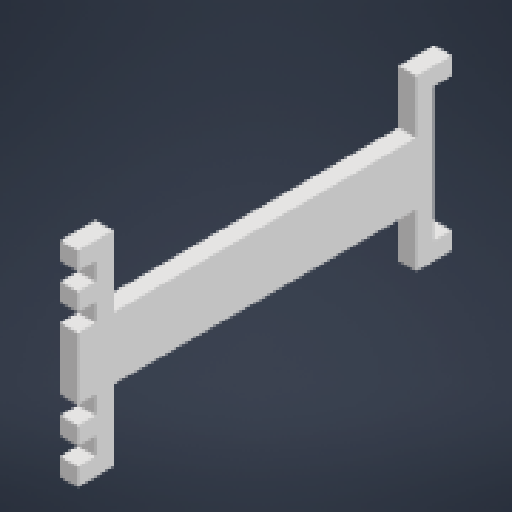
# Autodesk Inventor part: FootConnector
Saved by Autodesk Inventor 2027 (Build 310192000, 192)
## iProperties
Created: 2026-04-15
Part Number: FootConnector
Material: Generic
Document SubType Name: Modeling
Designer: Tueha
Density: 1 g/cm^3
Appearance: Default
Author: Tueha
Autodesk Inventor part; units mm, degrees
ref_plane "YZ Plane" through (0, 0, 0) normal (1, 0, 0) x (0, 1, 0)
ref_plane "XZ Plane" through (0, 0, 0) normal (0, 1, 0) x (-1, 0, 0)
ref_plane "XY Plane" through (0, 0, 0) normal (0, 0, 1) x (1, 0, 0)
sketch "Sketch1" plane through (0, 0, 0) normal (0, 0, 1) x (1, 0, 0)
  line L0 (316.5108, 23.0377) -> (310.3108, 23.0377) projected
  line L1 (316.5108, 39.9377) -> (316.5108, 23.0377) projected
  line L2 (316.5108, 39.9377) -> (24.9108, 39.9377) projected
  line L3 (24.9108, 39.9377) -> (24.9108, 45.9377) projected
  line L4 (24.9108, 45.9377) -> (316.5108, 45.9377) projected
  line L5 (316.5108, 62.8377) -> (316.5108, 45.9377) projected
  line L6 (301.1069, 62.8377) -> (316.5108, 62.8377) projected
  line L7 (295.9108, 65.8377) -> (301.1069, 62.8377) projected
  line L8 (295.9108, 62.8377) -> (295.9108, 65.8377) projected
  arc A0 (293.9108, 62.8377) -> (295.9108, 62.8377) centre (294.9108, 62.8377) ccw projected
  line L9 (293.9108, 65.8377) -> (293.9108, 62.8377) projected
  line L10 (288.7146, 62.8377) -> (293.9108, 65.8377) projected
  line L11 (272.3069, 62.8377) -> (288.7146, 62.8377) projected
  line L12 (267.1108, 65.8377) -> (272.3069, 62.8377) projected
  line L13 (267.1108, 62.8377) -> (267.1108, 65.8377) projected
  arc A1 (265.1108, 62.8377) -> (267.1108, 62.8377) centre (266.1108, 62.8377) ccw projected
  line L14 (265.1108, 65.8377) -> (265.1108, 62.8377) projected
  line L15 (259.9146, 62.8377) -> (265.1108, 65.8377) projected
  line L16 (243.5069, 62.8377) -> (259.9146, 62.8377) projected
  line L17 (238.3108, 65.8377) -> (243.5069, 62.8377) projected
  line L18 (238.3108, 62.8377) -> (238.3108, 65.8377) projected
  arc A2 (236.3108, 62.8377) -> (238.3108, 62.8377) centre (237.3108, 62.8377) ccw projected
  line L19 (236.3108, 65.8377) -> (236.3108, 62.8377) projected
  line L20 (231.1146, 62.8377) -> (236.3108, 65.8377) projected
  line L21 (214.7069, 62.8377) -> (231.1146, 62.8377) projected
  line L22 (209.5108, 65.8377) -> (214.7069, 62.8377) projected
  line L23 (209.5108, 62.8377) -> (209.5108, 65.8377) projected
  arc A3 (207.5108, 62.8377) -> (209.5108, 62.8377) centre (208.5108, 62.8377) ccw projected
  line L24 (207.5108, 65.8377) -> (207.5108, 62.8377) projected
  line L25 (202.3146, 62.8377) -> (207.5108, 65.8377) projected
  line L26 (185.9069, 62.8377) -> (202.3146, 62.8377) projected
  line L27 (180.7108, 65.8377) -> (185.9069, 62.8377) projected
  line L28 (180.7108, 62.8377) -> (180.7108, 65.8377) projected
  arc A4 (178.7108, 62.8377) -> (180.7108, 62.8377) centre (179.7108, 62.8377) ccw projected
  line L29 (178.7108, 65.8377) -> (178.7108, 62.8377) projected
  line L30 (173.5146, 62.8377) -> (178.7108, 65.8377) projected
  line L31 (157.1069, 62.8377) -> (173.5146, 62.8377) projected
  line L32 (151.9108, 65.8377) -> (157.1069, 62.8377) projected
  line L33 (151.9108, 62.8377) -> (151.9108, 65.8377) projected
  arc A5 (149.9108, 62.8377) -> (151.9108, 62.8377) centre (150.9108, 62.8377) ccw projected
  line L34 (149.9108, 65.8377) -> (149.9108, 62.8377) projected
  line L35 (144.7146, 62.8377) -> (149.9108, 65.8377) projected
  line L36 (128.3069, 62.8377) -> (144.7146, 62.8377) projected
  line L37 (123.1108, 65.8377) -> (128.3069, 62.8377) projected
  line L38 (123.1108, 62.8377) -> (123.1108, 65.8377) projected
  arc A6 (121.1108, 62.8377) -> (123.1108, 62.8377) centre (122.1108, 62.8377) ccw projected
  line L39 (121.1108, 65.8377) -> (121.1108, 62.8377) projected
  line L40 (115.9146, 62.8377) -> (121.1108, 65.8377) projected
  line L41 (99.5069, 62.8377) -> (115.9146, 62.8377) projected
  line L42 (94.3108, 65.8377) -> (99.5069, 62.8377) projected
  line L43 (94.3108, 62.8377) -> (94.3108, 65.8377) projected
  arc A7 (92.3108, 62.8377) -> (94.3108, 62.8377) centre (93.3108, 62.8377) ccw projected
  line L44 (92.3108, 65.8377) -> (92.3108, 62.8377) projected
  line L45 (87.1146, 62.8377) -> (92.3108, 65.8377) projected
  line L46 (70.7069, 62.8377) -> (87.1146, 62.8377) projected
  line L47 (65.5108, 65.8377) -> (70.7069, 62.8377) projected
  line L48 (65.5108, 62.8377) -> (65.5108, 65.8377) projected
  arc A8 (63.5108, 62.8377) -> (65.5108, 62.8377) centre (64.5108, 62.8377) ccw projected
  line L49 (63.5108, 65.8377) -> (63.5108, 62.8377) projected
  line L50 (58.3146, 62.8377) -> (63.5108, 65.8377) projected
  line L51 (41.9069, 62.8377) -> (58.3146, 62.8377) projected
  line L52 (36.7108, 65.8377) -> (41.9069, 62.8377) projected
  line L53 (36.7108, 62.8377) -> (36.7108, 65.8377) projected
  arc A9 (34.7108, 62.8377) -> (36.7108, 62.8377) centre (35.7108, 62.8377) ccw projected
  line L54 (34.7108, 65.8377) -> (34.7108, 62.8377) projected
  line L55 (29.5146, 62.8377) -> (34.7108, 65.8377) projected
  line L56 (13.1069, 62.8377) -> (29.5146, 62.8377) projected
  line L57 (7.9108, 65.8377) -> (13.1069, 62.8377) projected
  line L58 (7.9108, 62.8377) -> (7.9108, 65.8377) projected
  arc A10 (5.9108, 62.8377) -> (7.9108, 62.8377) centre (6.9108, 62.8377) ccw projected
  line L59 (5.9108, 65.8377) -> (5.9108, 62.8377) projected
  line L60 (0.7146, 62.8377) -> (5.9108, 65.8377) projected
  line L61 (-15.6931, 62.8377) -> (0.7146, 62.8377) projected
  line L62 (-20.8892, 65.8377) -> (-15.6931, 62.8377) projected
  line L63 (-20.8892, 62.8377) -> (-20.8892, 65.8377) projected
  arc A11 (-22.8892, 62.8377) -> (-20.8892, 62.8377) centre (-21.8892, 62.8377) ccw projected
  line L64 (-22.8892, 65.8377) -> (-22.8892, 62.8377) projected
  line L65 (-28.0854, 62.8377) -> (-22.8892, 65.8377) projected
  line L66 (-44.4931, 62.8377) -> (-28.0854, 62.8377) projected
  line L67 (-49.6892, 65.8377) -> (-44.4931, 62.8377) projected
  line L68 (-49.6892, 62.8377) -> (-49.6892, 65.8377) projected
  arc A12 (-51.6892, 62.8377) -> (-49.6892, 62.8377) centre (-50.6892, 62.8377) ccw projected
  line L69 (-51.6892, 65.8377) -> (-51.6892, 62.8377) projected
  line L70 (-56.8854, 62.8377) -> (-51.6892, 65.8377) projected
  line L71 (-73.2931, 62.8377) -> (-56.8854, 62.8377) projected
  line L72 (-78.4892, 65.8377) -> (-73.2931, 62.8377) projected
  line L73 (-78.4892, 62.8377) -> (-78.4892, 65.8377) projected
  arc A13 (-80.4892, 62.8377) -> (-78.4892, 62.8377) centre (-79.4892, 62.8377) ccw projected
  line L74 (-80.4892, 65.8377) -> (-80.4892, 62.8377) projected
  line L75 (-85.6854, 62.8377) -> (-80.4892, 65.8377) projected
  line L76 (-102.0931, 62.8377) -> (-85.6854, 62.8377) projected
  line L77 (-107.2892, 65.8377) -> (-102.0931, 62.8377) projected
  line L78 (-107.2892, 62.8377) -> (-107.2892, 65.8377) projected
  arc A14 (-109.2892, 62.8377) -> (-107.2892, 62.8377) centre (-108.2892, 62.8377) ccw projected
  line L79 (-109.2892, 65.8377) -> (-109.2892, 62.8377) projected
  line L80 (-114.4854, 62.8377) -> (-109.2892, 65.8377) projected
  line L81 (-130.8931, 62.8377) -> (-114.4854, 62.8377) projected
  line L82 (-136.0892, 65.8377) -> (-130.8931, 62.8377) projected
  line L83 (-136.0892, 62.8377) -> (-136.0892, 65.8377) projected
  arc A15 (-138.0892, 62.8377) -> (-136.0892, 62.8377) centre (-137.0892, 62.8377) ccw projected
  line L84 (-138.0892, 65.8377) -> (-138.0892, 62.8377) projected
  line L85 (-143.2854, 62.8377) -> (-138.0892, 65.8377) projected
  line L86 (-159.6931, 62.8377) -> (-143.2854, 62.8377) projected
  line L87 (-164.8892, 65.8377) -> (-159.6931, 62.8377) projected
  line L88 (-164.8892, 62.8377) -> (-164.8892, 65.8377) projected
  arc A16 (-166.8892, 62.8377) -> (-164.8892, 62.8377) centre (-165.8892, 62.8377) ccw projected
  line L89 (-166.8892, 65.8377) -> (-166.8892, 62.8377) projected
  line L90 (-172.0854, 62.8377) -> (-166.8892, 65.8377) projected
  line L91 (-188.4931, 62.8377) -> (-172.0854, 62.8377) projected
  line L92 (-193.6892, 65.8377) -> (-188.4931, 62.8377) projected
  line L93 (-193.6892, 62.8377) -> (-193.6892, 65.8377) projected
  arc A17 (-195.6892, 62.8377) -> (-193.6892, 62.8377) centre (-194.6892, 62.8377) ccw projected
  line L94 (-195.6892, 65.8377) -> (-195.6892, 62.8377) projected
  line L95 (-200.8854, 62.8377) -> (-195.6892, 65.8377) projected
  line L96 (-217.2931, 62.8377) -> (-200.8854, 62.8377) projected
  line L97 (-222.4892, 65.8377) -> (-217.2931, 62.8377) projected
  line L98 (-222.4892, 62.8377) -> (-222.4892, 65.8377) projected
  arc A18 (-224.4892, 62.8377) -> (-222.4892, 62.8377) centre (-223.4892, 62.8377) ccw projected
  line L99 (-224.4892, 65.8377) -> (-224.4892, 62.8377) projected
  line L100 (-229.6854, 62.8377) -> (-224.4892, 65.8377) projected
  line L101 (-246.0931, 62.8377) -> (-229.6854, 62.8377) projected
  line L102 (-251.2892, 65.8377) -> (-246.0931, 62.8377) projected
  line L103 (-251.2892, 62.8377) -> (-251.2892, 65.8377) projected
  arc A19 (-253.2892, 62.8377) -> (-251.2892, 62.8377) centre (-252.2892, 62.8377) ccw projected
  line L104 (-253.2892, 65.8377) -> (-253.2892, 62.8377) projected
  line L105 (-258.4854, 62.8377) -> (-253.2892, 65.8377) projected
  line L106 (-258.4854, 62.8377) -> (-266.6892, 62.8377) projected
  line L107 (-266.6892, 23.0377) -> (-266.6892, 62.8377) projected
  line L108 (-244.0854, 23.0377) -> (-266.6892, 23.0377) projected
  line L109 (-238.8892, 20.0377) -> (-244.0854, 23.0377) projected
  line L110 (-238.8892, 23.0377) -> (-238.8892, 20.0377) projected
  arc A20 (-236.8892, 23.0377) -> (-238.8892, 23.0377) centre (-237.8892, 23.0377) ccw projected
  line L111 (-236.8892, 20.0377) -> (-236.8892, 23.0377) projected
  line L112 (-231.6931, 23.0377) -> (-236.8892, 20.0377) projected
  line L113 (-215.2854, 23.0377) -> (-231.6931, 23.0377) projected
  line L114 (-210.0892, 20.0377) -> (-215.2854, 23.0377) projected
  line L115 (-210.0892, 23.0377) -> (-210.0892, 20.0377) projected
  arc A21 (-208.0892, 23.0377) -> (-210.0892, 23.0377) centre (-209.0892, 23.0377) ccw projected
  line L116 (-208.0892, 20.0377) -> (-208.0892, 23.0377) projected
  line L117 (-202.8931, 23.0377) -> (-208.0892, 20.0377) projected
  line L118 (-186.4854, 23.0377) -> (-202.8931, 23.0377) projected
  line L119 (-181.2892, 20.0377) -> (-186.4854, 23.0377) projected
  line L120 (-181.2892, 23.0377) -> (-181.2892, 20.0377) projected
  arc A22 (-179.2892, 23.0377) -> (-181.2892, 23.0377) centre (-180.2892, 23.0377) ccw projected
  line L121 (-179.2892, 20.0377) -> (-179.2892, 23.0377) projected
  line L122 (-174.0931, 23.0377) -> (-179.2892, 20.0377) projected
  line L123 (-157.6854, 23.0377) -> (-174.0931, 23.0377) projected
  line L124 (-152.4892, 20.0377) -> (-157.6854, 23.0377) projected
  line L125 (-152.4892, 23.0377) -> (-152.4892, 20.0377) projected
  arc A23 (-150.4892, 23.0377) -> (-152.4892, 23.0377) centre (-151.4892, 23.0377) ccw projected
  line L126 (-150.4892, 20.0377) -> (-150.4892, 23.0377) projected
  line L127 (-145.2931, 23.0377) -> (-150.4892, 20.0377) projected
  line L128 (-128.8854, 23.0377) -> (-145.2931, 23.0377) projected
  line L129 (-123.6892, 20.0377) -> (-128.8854, 23.0377) projected
  line L130 (-123.6892, 23.0377) -> (-123.6892, 20.0377) projected
  arc A24 (-121.6892, 23.0377) -> (-123.6892, 23.0377) centre (-122.6892, 23.0377) ccw projected
  line L131 (-121.6892, 20.0377) -> (-121.6892, 23.0377) projected
  line L132 (-116.4931, 23.0377) -> (-121.6892, 20.0377) projected
  line L133 (-100.0854, 23.0377) -> (-116.4931, 23.0377) projected
  line L134 (-94.8892, 20.0377) -> (-100.0854, 23.0377) projected
  line L135 (-94.8892, 23.0377) -> (-94.8892, 20.0377) projected
  arc A25 (-92.8892, 23.0377) -> (-94.8892, 23.0377) centre (-93.8892, 23.0377) ccw projected
  line L136 (-92.8892, 20.0377) -> (-92.8892, 23.0377) projected
  line L137 (-87.6931, 23.0377) -> (-92.8892, 20.0377) projected
  line L138 (-71.2854, 23.0377) -> (-87.6931, 23.0377) projected
  line L139 (-66.0892, 20.0377) -> (-71.2854, 23.0377) projected
  line L140 (-66.0892, 23.0377) -> (-66.0892, 20.0377) projected
  arc A26 (-64.0892, 23.0377) -> (-66.0892, 23.0377) centre (-65.0892, 23.0377) ccw projected
  line L141 (-64.0892, 20.0377) -> (-64.0892, 23.0377) projected
  line L142 (-58.8931, 23.0377) -> (-64.0892, 20.0377) projected
  line L143 (-42.4854, 23.0377) -> (-58.8931, 23.0377) projected
  line L144 (-37.2892, 20.0377) -> (-42.4854, 23.0377) projected
  line L145 (-37.2892, 23.0377) -> (-37.2892, 20.0377) projected
  arc A27 (-35.2892, 23.0377) -> (-37.2892, 23.0377) centre (-36.2892, 23.0377) ccw projected
  line L146 (-35.2892, 20.0377) -> (-35.2892, 23.0377) projected
  line L147 (-30.0931, 23.0377) -> (-35.2892, 20.0377) projected
  line L148 (-13.6854, 23.0377) -> (-30.0931, 23.0377) projected
  line L149 (-8.4892, 20.0377) -> (-13.6854, 23.0377) projected
  line L150 (-8.4892, 23.0377) -> (-8.4892, 20.0377) projected
  arc A28 (-6.4892, 23.0377) -> (-8.4892, 23.0377) centre (-7.4892, 23.0377) ccw projected
  line L151 (-6.4892, 20.0377) -> (-6.4892, 23.0377) projected
  line L152 (-1.2931, 23.0377) -> (-6.4892, 20.0377) projected
  line L153 (15.1146, 23.0377) -> (-1.2931, 23.0377) projected
  line L154 (20.3108, 20.0377) -> (15.1146, 23.0377) projected
  line L155 (20.3108, 23.0377) -> (20.3108, 20.0377) projected
  arc A29 (22.3108, 23.0377) -> (20.3108, 23.0377) centre (21.3108, 23.0377) ccw projected
  line L156 (22.3108, 20.0377) -> (22.3108, 23.0377) projected
  line L157 (27.5069, 23.0377) -> (22.3108, 20.0377) projected
  line L158 (43.9146, 23.0377) -> (27.5069, 23.0377) projected
  line L159 (49.1108, 20.0377) -> (43.9146, 23.0377) projected
  line L160 (49.1108, 23.0377) -> (49.1108, 20.0377) projected
  arc A30 (51.1108, 23.0377) -> (49.1108, 23.0377) centre (50.1108, 23.0377) ccw projected
  line L161 (51.1108, 20.0377) -> (51.1108, 23.0377) projected
  line L162 (56.3069, 23.0377) -> (51.1108, 20.0377) projected
  line L163 (72.7146, 23.0377) -> (56.3069, 23.0377) projected
  line L164 (77.9108, 20.0377) -> (72.7146, 23.0377) projected
  line L165 (77.9108, 23.0377) -> (77.9108, 20.0377) projected
  arc A31 (79.9108, 23.0377) -> (77.9108, 23.0377) centre (78.9108, 23.0377) ccw projected
  line L166 (79.9108, 20.0377) -> (79.9108, 23.0377) projected
  line L167 (85.1069, 23.0377) -> (79.9108, 20.0377) projected
  line L168 (101.5146, 23.0377) -> (85.1069, 23.0377) projected
  line L169 (106.7108, 20.0377) -> (101.5146, 23.0377) projected
  line L170 (106.7108, 23.0377) -> (106.7108, 20.0377) projected
  arc A32 (108.7108, 23.0377) -> (106.7108, 23.0377) centre (107.7108, 23.0377) ccw projected
  line L171 (108.7108, 20.0377) -> (108.7108, 23.0377) projected
  line L172 (113.9069, 23.0377) -> (108.7108, 20.0377) projected
  line L173 (130.3146, 23.0377) -> (113.9069, 23.0377) projected
  line L174 (135.5108, 20.0377) -> (130.3146, 23.0377) projected
  line L175 (135.5108, 23.0377) -> (135.5108, 20.0377) projected
  arc A33 (137.5108, 23.0377) -> (135.5108, 23.0377) centre (136.5108, 23.0377) ccw projected
  line L176 (137.5108, 20.0377) -> (137.5108, 23.0377) projected
  line L177 (142.7069, 23.0377) -> (137.5108, 20.0377) projected
  line L178 (159.1146, 23.0377) -> (142.7069, 23.0377) projected
  line L179 (164.3108, 20.0377) -> (159.1146, 23.0377) projected
  line L180 (164.3108, 23.0377) -> (164.3108, 20.0377) projected
  arc A34 (166.3108, 23.0377) -> (164.3108, 23.0377) centre (165.3108, 23.0377) ccw projected
  line L181 (166.3108, 20.0377) -> (166.3108, 23.0377) projected
  line L182 (171.5069, 23.0377) -> (166.3108, 20.0377) projected
  line L183 (187.9146, 23.0377) -> (171.5069, 23.0377) projected
  line L184 (193.1108, 20.0377) -> (187.9146, 23.0377) projected
  line L185 (193.1108, 23.0377) -> (193.1108, 20.0377) projected
  arc A35 (195.1108, 23.0377) -> (193.1108, 23.0377) centre (194.1108, 23.0377) ccw projected
  line L186 (195.1108, 20.0377) -> (195.1108, 23.0377) projected
  line L187 (200.3069, 23.0377) -> (195.1108, 20.0377) projected
  line L188 (216.7146, 23.0377) -> (200.3069, 23.0377) projected
  line L189 (221.9108, 20.0377) -> (216.7146, 23.0377) projected
  line L190 (221.9108, 23.0377) -> (221.9108, 20.0377) projected
  arc A36 (223.9108, 23.0377) -> (221.9108, 23.0377) centre (222.9108, 23.0377) ccw projected
  line L191 (223.9108, 20.0377) -> (223.9108, 23.0377) projected
  line L192 (229.1069, 23.0377) -> (223.9108, 20.0377) projected
  line L193 (245.5146, 23.0377) -> (229.1069, 23.0377) projected
  line L194 (250.7108, 20.0377) -> (245.5146, 23.0377) projected
  line L195 (250.7108, 23.0377) -> (250.7108, 20.0377) projected
  arc A37 (252.7108, 23.0377) -> (250.7108, 23.0377) centre (251.7108, 23.0377) ccw projected
  line L196 (252.7108, 20.0377) -> (252.7108, 23.0377) projected
  line L197 (257.9069, 23.0377) -> (252.7108, 20.0377) projected
  line L198 (274.3146, 23.0377) -> (257.9069, 23.0377) projected
  line L199 (279.5108, 20.0377) -> (274.3146, 23.0377) projected
  line L200 (279.5108, 23.0377) -> (279.5108, 20.0377) projected
  arc A38 (281.5108, 23.0377) -> (279.5108, 23.0377) centre (280.5108, 23.0377) ccw projected
  line L201 (281.5108, 20.0377) -> (281.5108, 23.0377) projected
  line L202 (286.7069, 23.0377) -> (281.5108, 20.0377) projected
  line L203 (303.1146, 23.0377) -> (286.7069, 23.0377) projected
  line L204 (308.3108, 20.0377) -> (303.1146, 23.0377) projected
  line L205 (308.3108, 23.0377) -> (308.3108, 20.0377) projected
  arc A39 (310.3108, 23.0377) -> (308.3108, 23.0377) centre (309.3108, 23.0377) ccw projected
  line L206 (-237.2892, 33.9377) -> (-231.2892, 33.9377) projected
  line L207 (-231.2892, 33.9377) -> (-231.2892, 27.9377) projected
  line L208 (-231.2892, 27.9377) -> (-237.2892, 27.9377) projected
  line L209 (-237.2892, 27.9377) -> (-237.2892, 33.9377) projected
  line L210 (-237.2892, 51.9377) -> (-237.2892, 57.9377) projected
  line L211 (-237.2892, 57.9377) -> (-231.2892, 57.9377) projected
  line L212 (-231.2892, 57.9377) -> (-231.2892, 51.9377) projected
  line L213 (-231.2892, 51.9377) -> (-237.2892, 51.9377) projected
  line L214 (-179.6892, 33.9377) -> (-173.6892, 33.9377) projected
  line L215 (-173.6892, 33.9377) -> (-173.6892, 27.9377) projected
  line L216 (-173.6892, 27.9377) -> (-179.6892, 27.9377) projected
  line L217 (-179.6892, 27.9377) -> (-179.6892, 33.9377) projected
  line L218 (-179.6892, 51.9377) -> (-179.6892, 57.9377) projected
  line L219 (-179.6892, 57.9377) -> (-173.6892, 57.9377) projected
  line L220 (-173.6892, 57.9377) -> (-173.6892, 51.9377) projected
  line L221 (-173.6892, 51.9377) -> (-179.6892, 51.9377) projected
  line L222 (-122.0892, 33.9377) -> (-116.0892, 33.9377) projected
  line L223 (-116.0892, 33.9377) -> (-116.0892, 27.9377) projected
  line L224 (-116.0892, 27.9377) -> (-122.0892, 27.9377) projected
  line L225 (-122.0892, 27.9377) -> (-122.0892, 33.9377) projected
  line L226 (-122.0892, 51.9377) -> (-122.0892, 57.9377) projected
  line L227 (-122.0892, 57.9377) -> (-116.0892, 57.9377) projected
  line L228 (-116.0892, 57.9377) -> (-116.0892, 51.9377) projected
  line L229 (-116.0892, 51.9377) -> (-122.0892, 51.9377) projected
  line L230 (-64.4892, 33.9377) -> (-58.4892, 33.9377) projected
  line L231 (-58.4892, 33.9377) -> (-58.4892, 27.9377) projected
  line L232 (-58.4892, 27.9377) -> (-64.4892, 27.9377) projected
  line L233 (-64.4892, 27.9377) -> (-64.4892, 33.9377) projected
  line L234 (-64.4892, 51.9377) -> (-64.4892, 57.9377) projected
  line L235 (-64.4892, 57.9377) -> (-58.4892, 57.9377) projected
  line L236 (-58.4892, 57.9377) -> (-58.4892, 51.9377) projected
  line L237 (-58.4892, 51.9377) -> (-64.4892, 51.9377) projected
  line L238 (-6.8892, 33.9377) -> (-0.8892, 33.9377) projected
  line L239 (-0.8892, 33.9377) -> (-0.8892, 27.9377) projected
  line L240 (-0.8892, 27.9377) -> (-6.8892, 27.9377) projected
  line L241 (-6.8892, 27.9377) -> (-6.8892, 33.9377) projected
  line L242 (-6.8892, 51.9377) -> (-6.8892, 57.9377) projected
  line L243 (-6.8892, 57.9377) -> (-0.8892, 57.9377) projected
  line L244 (-0.8892, 57.9377) -> (-0.8892, 51.9377) projected
  line L245 (-0.8892, 51.9377) -> (-6.8892, 51.9377) projected
  line L246 (50.7108, 33.9377) -> (56.7108, 33.9377) projected
  line L247 (56.7108, 33.9377) -> (56.7108, 27.9377) projected
  line L248 (56.7108, 27.9377) -> (50.7108, 27.9377) projected
  line L249 (50.7108, 27.9377) -> (50.7108, 33.9377) projected
  line L250 (50.7108, 51.9377) -> (50.7108, 57.9377) projected
  line L251 (50.7108, 57.9377) -> (56.7108, 57.9377) projected
  line L252 (56.7108, 57.9377) -> (56.7108, 51.9377) projected
  line L253 (56.7108, 51.9377) -> (50.7108, 51.9377) projected
  line L254 (108.3108, 33.9377) -> (114.3108, 33.9377) projected
  line L255 (114.3108, 33.9377) -> (114.3108, 27.9377) projected
  line L256 (114.3108, 27.9377) -> (108.3108, 27.9377) projected
  line L257 (108.3108, 27.9377) -> (108.3108, 33.9377) projected
  line L258 (108.3108, 51.9377) -> (108.3108, 57.9377) projected
  line L259 (108.3108, 57.9377) -> (114.3108, 57.9377) projected
  line L260 (114.3108, 57.9377) -> (114.3108, 51.9377) projected
  line L261 (114.3108, 51.9377) -> (108.3108, 51.9377) projected
  line L262 (165.9108, 33.9377) -> (171.9108, 33.9377) projected
  line L263 (171.9108, 33.9377) -> (171.9108, 27.9377) projected
  line L264 (171.9108, 27.9377) -> (165.9108, 27.9377) projected
  line L265 (165.9108, 27.9377) -> (165.9108, 33.9377) projected
  line L266 (165.9108, 51.9377) -> (165.9108, 57.9377) projected
  line L267 (165.9108, 57.9377) -> (171.9108, 57.9377) projected
  line L268 (171.9108, 57.9377) -> (171.9108, 51.9377) projected
  line L269 (171.9108, 51.9377) -> (165.9108, 51.9377) projected
  line L270 (223.5108, 33.9377) -> (229.5108, 33.9377) projected
  line L271 (229.5108, 33.9377) -> (229.5108, 27.9377) projected
  line L272 (229.5108, 27.9377) -> (223.5108, 27.9377) projected
  line L273 (223.5108, 27.9377) -> (223.5108, 33.9377) projected
  line L274 (223.5108, 51.9377) -> (223.5108, 57.9377) projected
  line L275 (223.5108, 57.9377) -> (229.5108, 57.9377) projected
  line L276 (229.5108, 57.9377) -> (229.5108, 51.9377) projected
  line L277 (229.5108, 51.9377) -> (223.5108, 51.9377) projected
  line L278 (281.1108, 33.9377) -> (287.1108, 33.9377) projected
  line L279 (287.1108, 33.9377) -> (287.1108, 27.9377) projected
  line L280 (287.1108, 27.9377) -> (281.1108, 27.9377) projected
  line L281 (281.1108, 27.9377) -> (281.1108, 33.9377) projected
  line L282 (281.1108, 51.9377) -> (281.1108, 57.9377) projected
  line L283 (281.1108, 57.9377) -> (287.1108, 57.9377) projected
  line L284 (287.1108, 57.9377) -> (287.1108, 51.9377) projected
  line L285 (287.1108, 51.9377) -> (281.1108, 51.9377) projected
  line L286 (316.5108, -51.9623) -> (310.3108, -51.9623) projected
  line L287 (316.5108, -35.0623) -> (316.5108, -51.9623) projected
  line L288 (316.5108, -35.0623) -> (24.9108, -35.0623) projected
  line L289 (24.9108, -35.0623) -> (24.9108, -29.0623) projected
  line L290 (24.9108, -29.0623) -> (316.5108, -29.0623) projected
  line L291 (316.5108, -12.1623) -> (316.5108, -29.0623) projected
  line L292 (301.1069, -12.1623) -> (316.5108, -12.1623) projected
  line L293 (295.9108, -9.1623) -> (301.1069, -12.1623) projected
  line L294 (295.9108, -12.1623) -> (295.9108, -9.1623) projected
  arc A40 (293.9108, -12.1623) -> (295.9108, -12.1623) centre (294.9108, -12.1623) ccw projected
  line L295 (293.9108, -9.1623) -> (293.9108, -12.1623) projected
  line L296 (288.7146, -12.1623) -> (293.9108, -9.1623) projected
  line L297 (272.3069, -12.1623) -> (288.7146, -12.1623) projected
  line L298 (267.1108, -9.1623) -> (272.3069, -12.1623) projected
  line L299 (267.1108, -12.1623) -> (267.1108, -9.1623) projected
  arc A41 (265.1108, -12.1623) -> (267.1108, -12.1623) centre (266.1108, -12.1623) ccw projected
  line L300 (265.1108, -9.1623) -> (265.1108, -12.1623) projected
  line L301 (259.9146, -12.1623) -> (265.1108, -9.1623) projected
  line L302 (243.5069, -12.1623) -> (259.9146, -12.1623) projected
  line L303 (238.3108, -9.1623) -> (243.5069, -12.1623) projected
  line L304 (238.3108, -12.1623) -> (238.3108, -9.1623) projected
  arc A42 (236.3108, -12.1623) -> (238.3108, -12.1623) centre (237.3108, -12.1623) ccw projected
  line L305 (236.3108, -9.1623) -> (236.3108, -12.1623) projected
  line L306 (231.1146, -12.1623) -> (236.3108, -9.1623) projected
  line L307 (214.7069, -12.1623) -> (231.1146, -12.1623) projected
  line L308 (209.5108, -9.1623) -> (214.7069, -12.1623) projected
  line L309 (209.5108, -12.1623) -> (209.5108, -9.1623) projected
  arc A43 (207.5108, -12.1623) -> (209.5108, -12.1623) centre (208.5108, -12.1623) ccw projected
  line L310 (207.5108, -9.1623) -> (207.5108, -12.1623) projected
  line L311 (202.3146, -12.1623) -> (207.5108, -9.1623) projected
  line L312 (185.9069, -12.1623) -> (202.3146, -12.1623) projected
  line L313 (180.7108, -9.1623) -> (185.9069, -12.1623) projected
  line L314 (180.7108, -12.1623) -> (180.7108, -9.1623) projected
  arc A44 (178.7108, -12.1623) -> (180.7108, -12.1623) centre (179.7108, -12.1623) ccw projected
  line L315 (178.7108, -9.1623) -> (178.7108, -12.1623) projected
  line L316 (173.5146, -12.1623) -> (178.7108, -9.1623) projected
  line L317 (157.1069, -12.1623) -> (173.5146, -12.1623) projected
  line L318 (151.9108, -9.1623) -> (157.1069, -12.1623) projected
  line L319 (151.9108, -12.1623) -> (151.9108, -9.1623) projected
  arc A45 (149.9108, -12.1623) -> (151.9108, -12.1623) centre (150.9108, -12.1623) ccw projected
  line L320 (149.9108, -9.1623) -> (149.9108, -12.1623) projected
  line L321 (144.7146, -12.1623) -> (149.9108, -9.1623) projected
  line L322 (128.3069, -12.1623) -> (144.7146, -12.1623) projected
  line L323 (123.1108, -9.1623) -> (128.3069, -12.1623) projected
  line L324 (123.1108, -12.1623) -> (123.1108, -9.1623) projected
  arc A46 (121.1108, -12.1623) -> (123.1108, -12.1623) centre (122.1108, -12.1623) ccw projected
  line L325 (121.1108, -9.1623) -> (121.1108, -12.1623) projected
  line L326 (115.9146, -12.1623) -> (121.1108, -9.1623) projected
  line L327 (99.5069, -12.1623) -> (115.9146, -12.1623) projected
  line L328 (94.3108, -9.1623) -> (99.5069, -12.1623) projected
  line L329 (94.3108, -12.1623) -> (94.3108, -9.1623) projected
  arc A47 (92.3108, -12.1623) -> (94.3108, -12.1623) centre (93.3108, -12.1623) ccw projected
  line L330 (92.3108, -9.1623) -> (92.3108, -12.1623) projected
  line L331 (87.1146, -12.1623) -> (92.3108, -9.1623) projected
  line L332 (70.7069, -12.1623) -> (87.1146, -12.1623) projected
  line L333 (65.5108, -9.1623) -> (70.7069, -12.1623) projected
  line L334 (65.5108, -12.1623) -> (65.5108, -9.1623) projected
  arc A48 (63.5108, -12.1623) -> (65.5108, -12.1623) centre (64.5108, -12.1623) ccw projected
  line L335 (63.5108, -9.1623) -> (63.5108, -12.1623) projected
  line L336 (58.3146, -12.1623) -> (63.5108, -9.1623) projected
  line L337 (41.9069, -12.1623) -> (58.3146, -12.1623) projected
  line L338 (36.7108, -9.1623) -> (41.9069, -12.1623) projected
  line L339 (36.7108, -12.1623) -> (36.7108, -9.1623) projected
  arc A49 (34.7108, -12.1623) -> (36.7108, -12.1623) centre (35.7108, -12.1623) ccw projected
  line L340 (34.7108, -9.1623) -> (34.7108, -12.1623) projected
  line L341 (29.5146, -12.1623) -> (34.7108, -9.1623) projected
  line L342 (13.1069, -12.1623) -> (29.5146, -12.1623) projected
  line L343 (7.9108, -9.1623) -> (13.1069, -12.1623) projected
  line L344 (7.9108, -12.1623) -> (7.9108, -9.1623) projected
  arc A50 (5.9108, -12.1623) -> (7.9108, -12.1623) centre (6.9108, -12.1623) ccw projected
  line L345 (5.9108, -9.1623) -> (5.9108, -12.1623) projected
  line L346 (0.7146, -12.1623) -> (5.9108, -9.1623) projected
  line L347 (-15.6931, -12.1623) -> (0.7146, -12.1623) projected
  line L348 (-20.8892, -9.1623) -> (-15.6931, -12.1623) projected
  line L349 (-20.8892, -12.1623) -> (-20.8892, -9.1623) projected
  arc A51 (-22.8892, -12.1623) -> (-20.8892, -12.1623) centre (-21.8892, -12.1623) ccw projected
  line L350 (-22.8892, -9.1623) -> (-22.8892, -12.1623) projected
  line L351 (-28.0854, -12.1623) -> (-22.8892, -9.1623) projected
  line L352 (-44.4931, -12.1623) -> (-28.0854, -12.1623) projected
  line L353 (-49.6892, -9.1623) -> (-44.4931, -12.1623) projected
  line L354 (-49.6892, -12.1623) -> (-49.6892, -9.1623) projected
  arc A52 (-51.6892, -12.1623) -> (-49.6892, -12.1623) centre (-50.6892, -12.1623) ccw projected
  line L355 (-51.6892, -9.1623) -> (-51.6892, -12.1623) projected
  line L356 (-56.8854, -12.1623) -> (-51.6892, -9.1623) projected
  line L357 (-73.2931, -12.1623) -> (-56.8854, -12.1623) projected
  line L358 (-78.4892, -9.1623) -> (-73.2931, -12.1623) projected
  line L359 (-78.4892, -12.1623) -> (-78.4892, -9.1623) projected
  arc A53 (-80.4892, -12.1623) -> (-78.4892, -12.1623) centre (-79.4892, -12.1623) ccw projected
  line L360 (-80.4892, -9.1623) -> (-80.4892, -12.1623) projected
  line L361 (-85.6854, -12.1623) -> (-80.4892, -9.1623) projected
  line L362 (-102.0931, -12.1623) -> (-85.6854, -12.1623) projected
  line L363 (-107.2892, -9.1623) -> (-102.0931, -12.1623) projected
  line L364 (-107.2892, -12.1623) -> (-107.2892, -9.1623) projected
  arc A54 (-109.2892, -12.1623) -> (-107.2892, -12.1623) centre (-108.2892, -12.1623) ccw projected
  line L365 (-109.2892, -9.1623) -> (-109.2892, -12.1623) projected
  line L366 (-114.4854, -12.1623) -> (-109.2892, -9.1623) projected
  line L367 (-130.8931, -12.1623) -> (-114.4854, -12.1623) projected
  line L368 (-136.0892, -9.1623) -> (-130.8931, -12.1623) projected
  line L369 (-136.0892, -12.1623) -> (-136.0892, -9.1623) projected
  arc A55 (-138.0892, -12.1623) -> (-136.0892, -12.1623) centre (-137.0892, -12.1623) ccw projected
  line L370 (-138.0892, -9.1623) -> (-138.0892, -12.1623) projected
  line L371 (-143.2854, -12.1623) -> (-138.0892, -9.1623) projected
  line L372 (-159.6931, -12.1623) -> (-143.2854, -12.1623) projected
  line L373 (-164.8892, -9.1623) -> (-159.6931, -12.1623) projected
  line L374 (-164.8892, -12.1623) -> (-164.8892, -9.1623) projected
  arc A56 (-166.8892, -12.1623) -> (-164.8892, -12.1623) centre (-165.8892, -12.1623) ccw projected
  line L375 (-166.8892, -9.1623) -> (-166.8892, -12.1623) projected
  line L376 (-172.0854, -12.1623) -> (-166.8892, -9.1623) projected
  line L377 (-188.4931, -12.1623) -> (-172.0854, -12.1623) projected
  line L378 (-193.6892, -9.1623) -> (-188.4931, -12.1623) projected
  line L379 (-193.6892, -12.1623) -> (-193.6892, -9.1623) projected
  arc A57 (-195.6892, -12.1623) -> (-193.6892, -12.1623) centre (-194.6892, -12.1623) ccw projected
  line L380 (-195.6892, -9.1623) -> (-195.6892, -12.1623) projected
  line L381 (-200.8854, -12.1623) -> (-195.6892, -9.1623) projected
  line L382 (-217.2931, -12.1623) -> (-200.8854, -12.1623) projected
  line L383 (-222.4892, -9.1623) -> (-217.2931, -12.1623) projected
  line L384 (-222.4892, -12.1623) -> (-222.4892, -9.1623) projected
  arc A58 (-224.4892, -12.1623) -> (-222.4892, -12.1623) centre (-223.4892, -12.1623) ccw projected
  line L385 (-224.4892, -9.1623) -> (-224.4892, -12.1623) projected
  line L386 (-229.6854, -12.1623) -> (-224.4892, -9.1623) projected
  line L387 (-246.0931, -12.1623) -> (-229.6854, -12.1623) projected
  line L388 (-251.2892, -9.1623) -> (-246.0931, -12.1623) projected
  line L389 (-251.2892, -12.1623) -> (-251.2892, -9.1623) projected
  arc A59 (-253.2892, -12.1623) -> (-251.2892, -12.1623) centre (-252.2892, -12.1623) ccw projected
  line L390 (-253.2892, -9.1623) -> (-253.2892, -12.1623) projected
  line L391 (-258.4854, -12.1623) -> (-253.2892, -9.1623) projected
  line L392 (-258.4854, -12.1623) -> (-266.6892, -12.1623) projected
  line L393 (-266.6892, -51.9623) -> (-266.6892, -12.1623) projected
  line L394 (-244.0854, -51.9623) -> (-266.6892, -51.9623) projected
  line L395 (-238.8892, -54.9623) -> (-244.0854, -51.9623) projected
  line L396 (-238.8892, -51.9623) -> (-238.8892, -54.9623) projected
  arc A60 (-236.8892, -51.9623) -> (-238.8892, -51.9623) centre (-237.8892, -51.9623) ccw projected
  line L397 (-236.8892, -54.9623) -> (-236.8892, -51.9623) projected
  line L398 (-231.6931, -51.9623) -> (-236.8892, -54.9623) projected
  line L399 (-215.2854, -51.9623) -> (-231.6931, -51.9623) projected
  line L400 (-210.0892, -54.9623) -> (-215.2854, -51.9623) projected
  line L401 (-210.0892, -51.9623) -> (-210.0892, -54.9623) projected
  arc A61 (-208.0892, -51.9623) -> (-210.0892, -51.9623) centre (-209.0892, -51.9623) ccw projected
  line L402 (-208.0892, -54.9623) -> (-208.0892, -51.9623) projected
  line L403 (-202.8931, -51.9623) -> (-208.0892, -54.9623) projected
  line L404 (-186.4854, -51.9623) -> (-202.8931, -51.9623) projected
  line L405 (-181.2892, -54.9623) -> (-186.4854, -51.9623) projected
  line L406 (-181.2892, -51.9623) -> (-181.2892, -54.9623) projected
  arc A62 (-179.2892, -51.9623) -> (-181.2892, -51.9623) centre (-180.2892, -51.9623) ccw projected
  line L407 (-179.2892, -54.9623) -> (-179.2892, -51.9623) projected
  line L408 (-174.0931, -51.9623) -> (-179.2892, -54.9623) projected
  line L409 (-157.6854, -51.9623) -> (-174.0931, -51.9623) projected
  line L410 (-152.4892, -54.9623) -> (-157.6854, -51.9623) projected
  line L411 (-152.4892, -51.9623) -> (-152.4892, -54.9623) projected
  arc A63 (-150.4892, -51.9623) -> (-152.4892, -51.9623) centre (-151.4892, -51.9623) ccw projected
  line L412 (-150.4892, -54.9623) -> (-150.4892, -51.9623) projected
  line L413 (-145.2931, -51.9623) -> (-150.4892, -54.9623) projected
  line L414 (-128.8854, -51.9623) -> (-145.2931, -51.9623) projected
  line L415 (-123.6892, -54.9623) -> (-128.8854, -51.9623) projected
  line L416 (-123.6892, -51.9623) -> (-123.6892, -54.9623) projected
  arc A64 (-121.6892, -51.9623) -> (-123.6892, -51.9623) centre (-122.6892, -51.9623) ccw projected
  line L417 (-121.6892, -54.9623) -> (-121.6892, -51.9623) projected
  line L418 (-116.4931, -51.9623) -> (-121.6892, -54.9623) projected
  line L419 (-100.0854, -51.9623) -> (-116.4931, -51.9623) projected
  line L420 (-94.8892, -54.9623) -> (-100.0854, -51.9623) projected
  line L421 (-94.8892, -51.9623) -> (-94.8892, -54.9623) projected
  arc A65 (-92.8892, -51.9623) -> (-94.8892, -51.9623) centre (-93.8892, -51.9623) ccw projected
  line L422 (-92.8892, -54.9623) -> (-92.8892, -51.9623) projected
  line L423 (-87.6931, -51.9623) -> (-92.8892, -54.9623) projected
  line L424 (-71.2854, -51.9623) -> (-87.6931, -51.9623) projected
  line L425 (-66.0892, -54.9623) -> (-71.2854, -51.9623) projected
  line L426 (-66.0892, -51.9623) -> (-66.0892, -54.9623) projected
  arc A66 (-64.0892, -51.9623) -> (-66.0892, -51.9623) centre (-65.0892, -51.9623) ccw projected
  line L427 (-64.0892, -54.9623) -> (-64.0892, -51.9623) projected
  line L428 (-58.8931, -51.9623) -> (-64.0892, -54.9623) projected
  line L429 (-42.4854, -51.9623) -> (-58.8931, -51.9623) projected
  line L430 (-37.2892, -54.9623) -> (-42.4854, -51.9623) projected
  line L431 (-37.2892, -51.9623) -> (-37.2892, -54.9623) projected
  arc A67 (-35.2892, -51.9623) -> (-37.2892, -51.9623) centre (-36.2892, -51.9623) ccw projected
  line L432 (-35.2892, -54.9623) -> (-35.2892, -51.9623) projected
  line L433 (-30.0931, -51.9623) -> (-35.2892, -54.9623) projected
  line L434 (-13.6854, -51.9623) -> (-30.0931, -51.9623) projected
  line L435 (-8.4892, -54.9623) -> (-13.6854, -51.9623) projected
  line L436 (-8.4892, -51.9623) -> (-8.4892, -54.9623) projected
  arc A68 (-6.4892, -51.9623) -> (-8.4892, -51.9623) centre (-7.4892, -51.9623) ccw projected
  line L437 (-6.4892, -54.9623) -> (-6.4892, -51.9623) projected
  line L438 (-1.2931, -51.9623) -> (-6.4892, -54.9623) projected
  line L439 (15.1146, -51.9623) -> (-1.2931, -51.9623) projected
  line L440 (20.3108, -54.9623) -> (15.1146, -51.9623) projected
  line L441 (20.3108, -51.9623) -> (20.3108, -54.9623) projected
  arc A69 (22.3108, -51.9623) -> (20.3108, -51.9623) centre (21.3108, -51.9623) ccw projected
  line L442 (22.3108, -54.9623) -> (22.3108, -51.9623) projected
  line L443 (27.5069, -51.9623) -> (22.3108, -54.9623) projected
  line L444 (43.9146, -51.9623) -> (27.5069, -51.9623) projected
  line L445 (49.1108, -54.9623) -> (43.9146, -51.9623) projected
  line L446 (49.1108, -51.9623) -> (49.1108, -54.9623) projected
  arc A70 (51.1108, -51.9623) -> (49.1108, -51.9623) centre (50.1108, -51.9623) ccw projected
  line L447 (51.1108, -54.9623) -> (51.1108, -51.9623) projected
  line L448 (56.3069, -51.9623) -> (51.1108, -54.9623) projected
  line L449 (72.7146, -51.9623) -> (56.3069, -51.9623) projected
  line L450 (77.9108, -54.9623) -> (72.7146, -51.9623) projected
  line L451 (77.9108, -51.9623) -> (77.9108, -54.9623) projected
  arc A71 (79.9108, -51.9623) -> (77.9108, -51.9623) centre (78.9108, -51.9623) ccw projected
  line L452 (79.9108, -54.9623) -> (79.9108, -51.9623) projected
  line L453 (85.1069, -51.9623) -> (79.9108, -54.9623) projected
  line L454 (101.5146, -51.9623) -> (85.1069, -51.9623) projected
  line L455 (106.7108, -54.9623) -> (101.5146, -51.9623) projected
  line L456 (106.7108, -51.9623) -> (106.7108, -54.9623) projected
  arc A72 (108.7108, -51.9623) -> (106.7108, -51.9623) centre (107.7108, -51.9623) ccw projected
  line L457 (108.7108, -54.9623) -> (108.7108, -51.9623) projected
  line L458 (113.9069, -51.9623) -> (108.7108, -54.9623) projected
  line L459 (130.3146, -51.9623) -> (113.9069, -51.9623) projected
  line L460 (135.5108, -54.9623) -> (130.3146, -51.9623) projected
  line L461 (135.5108, -51.9623) -> (135.5108, -54.9623) projected
  arc A73 (137.5108, -51.9623) -> (135.5108, -51.9623) centre (136.5108, -51.9623) ccw projected
  line L462 (137.5108, -54.9623) -> (137.5108, -51.9623) projected
  line L463 (142.7069, -51.9623) -> (137.5108, -54.9623) projected
  line L464 (159.1146, -51.9623) -> (142.7069, -51.9623) projected
  line L465 (164.3108, -54.9623) -> (159.1146, -51.9623) projected
  line L466 (164.3108, -51.9623) -> (164.3108, -54.9623) projected
  arc A74 (166.3108, -51.9623) -> (164.3108, -51.9623) centre (165.3108, -51.9623) ccw projected
  line L467 (166.3108, -54.9623) -> (166.3108, -51.9623) projected
  line L468 (171.5069, -51.9623) -> (166.3108, -54.9623) projected
  line L469 (187.9146, -51.9623) -> (171.5069, -51.9623) projected
  line L470 (193.1108, -54.9623) -> (187.9146, -51.9623) projected
  line L471 (193.1108, -51.9623) -> (193.1108, -54.9623) projected
  arc A75 (195.1108, -51.9623) -> (193.1108, -51.9623) centre (194.1108, -51.9623) ccw projected
  line L472 (195.1108, -54.9623) -> (195.1108, -51.9623) projected
  line L473 (200.3069, -51.9623) -> (195.1108, -54.9623) projected
  line L474 (216.7146, -51.9623) -> (200.3069, -51.9623) projected
  line L475 (221.9108, -54.9623) -> (216.7146, -51.9623) projected
  line L476 (221.9108, -51.9623) -> (221.9108, -54.9623) projected
  arc A76 (223.9108, -51.9623) -> (221.9108, -51.9623) centre (222.9108, -51.9623) ccw projected
  line L477 (223.9108, -54.9623) -> (223.9108, -51.9623) projected
  line L478 (229.1069, -51.9623) -> (223.9108, -54.9623) projected
  line L479 (245.5146, -51.9623) -> (229.1069, -51.9623) projected
  line L480 (250.7108, -54.9623) -> (245.5146, -51.9623) projected
  line L481 (250.7108, -51.9623) -> (250.7108, -54.9623) projected
  arc A77 (252.7108, -51.9623) -> (250.7108, -51.9623) centre (251.7108, -51.9623) ccw projected
  line L482 (252.7108, -54.9623) -> (252.7108, -51.9623) projected
  line L483 (257.9069, -51.9623) -> (252.7108, -54.9623) projected
  line L484 (274.3146, -51.9623) -> (257.9069, -51.9623) projected
  line L485 (279.5108, -54.9623) -> (274.3146, -51.9623) projected
  line L486 (279.5108, -51.9623) -> (279.5108, -54.9623) projected
  arc A78 (281.5108, -51.9623) -> (279.5108, -51.9623) centre (280.5108, -51.9623) ccw projected
  line L487 (281.5108, -54.9623) -> (281.5108, -51.9623) projected
  line L488 (286.7069, -51.9623) -> (281.5108, -54.9623) projected
  line L489 (303.1146, -51.9623) -> (286.7069, -51.9623) projected
  line L490 (308.3108, -54.9623) -> (303.1146, -51.9623) projected
  line L491 (308.3108, -51.9623) -> (308.3108, -54.9623) projected
  arc A79 (310.3108, -51.9623) -> (308.3108, -51.9623) centre (309.3108, -51.9623) ccw projected
  line L492 (-237.2892, -41.0623) -> (-231.2892, -41.0623) projected
  line L493 (-231.2892, -41.0623) -> (-231.2892, -47.0623) projected
  line L494 (-231.2892, -47.0623) -> (-237.2892, -47.0623) projected
  line L495 (-237.2892, -47.0623) -> (-237.2892, -41.0623) projected
  line L496 (-237.2892, -23.0623) -> (-237.2892, -17.0623) projected
  line L497 (-237.2892, -17.0623) -> (-231.2892, -17.0623) projected
  line L498 (-231.2892, -17.0623) -> (-231.2892, -23.0623) projected
  line L499 (-231.2892, -23.0623) -> (-237.2892, -23.0623) projected
  line L500 (-179.6892, -41.0623) -> (-173.6892, -41.0623) projected
  line L501 (-173.6892, -41.0623) -> (-173.6892, -47.0623) projected
  line L502 (-173.6892, -47.0623) -> (-179.6892, -47.0623) projected
  line L503 (-179.6892, -47.0623) -> (-179.6892, -41.0623) projected
  line L504 (-179.6892, -23.0623) -> (-179.6892, -17.0623) projected
  line L505 (-179.6892, -17.0623) -> (-173.6892, -17.0623) projected
  line L506 (-173.6892, -17.0623) -> (-173.6892, -23.0623) projected
  line L507 (-173.6892, -23.0623) -> (-179.6892, -23.0623) projected
  line L508 (-122.0892, -41.0623) -> (-116.0892, -41.0623) projected
  line L509 (-116.0892, -41.0623) -> (-116.0892, -47.0623) projected
  line L510 (-116.0892, -47.0623) -> (-122.0892, -47.0623) projected
  line L511 (-122.0892, -47.0623) -> (-122.0892, -41.0623) projected
  line L512 (-122.0892, -23.0623) -> (-122.0892, -17.0623) projected
  line L513 (-122.0892, -17.0623) -> (-116.0892, -17.0623) projected
  line L514 (-116.0892, -17.0623) -> (-116.0892, -23.0623) projected
  line L515 (-116.0892, -23.0623) -> (-122.0892, -23.0623) projected
  line L516 (-64.4892, -41.0623) -> (-58.4892, -41.0623) projected
  line L517 (-58.4892, -41.0623) -> (-58.4892, -47.0623) projected
  line L518 (-58.4892, -47.0623) -> (-64.4892, -47.0623) projected
  line L519 (-64.4892, -47.0623) -> (-64.4892, -41.0623) projected
  line L520 (-64.4892, -23.0623) -> (-64.4892, -17.0623) projected
  line L521 (-64.4892, -17.0623) -> (-58.4892, -17.0623) projected
  line L522 (-58.4892, -17.0623) -> (-58.4892, -23.0623) projected
  line L523 (-58.4892, -23.0623) -> (-64.4892, -23.0623) projected
  line L524 (-6.8892, -41.0623) -> (-0.8892, -41.0623) projected
  line L525 (-0.8892, -41.0623) -> (-0.8892, -47.0623) projected
  line L526 (-0.8892, -47.0623) -> (-6.8892, -47.0623) projected
  line L527 (-6.8892, -47.0623) -> (-6.8892, -41.0623) projected
  line L528 (-6.8892, -23.0623) -> (-6.8892, -17.0623) projected
  line L529 (-6.8892, -17.0623) -> (-0.8892, -17.0623) projected
  line L530 (-0.8892, -17.0623) -> (-0.8892, -23.0623) projected
  line L531 (-0.8892, -23.0623) -> (-6.8892, -23.0623) projected
  line L532 (50.7108, -41.0623) -> (56.7108, -41.0623) projected
  line L533 (56.7108, -41.0623) -> (56.7108, -47.0623) projected
  line L534 (56.7108, -47.0623) -> (50.7108, -47.0623) projected
  line L535 (50.7108, -47.0623) -> (50.7108, -41.0623) projected
  line L536 (50.7108, -23.0623) -> (50.7108, -17.0623) projected
  line L537 (50.7108, -17.0623) -> (56.7108, -17.0623) projected
  line L538 (56.7108, -17.0623) -> (56.7108, -23.0623) projected
  line L539 (56.7108, -23.0623) -> (50.7108, -23.0623) projected
  line L540 (108.3108, -41.0623) -> (114.3108, -41.0623) projected
  line L541 (114.3108, -41.0623) -> (114.3108, -47.0623) projected
  line L542 (114.3108, -47.0623) -> (108.3108, -47.0623) projected
  line L543 (108.3108, -47.0623) -> (108.3108, -41.0623) projected
  line L544 (108.3108, -23.0623) -> (108.3108, -17.0623) projected
  line L545 (108.3108, -17.0623) -> (114.3108, -17.0623) projected
  line L546 (114.3108, -17.0623) -> (114.3108, -23.0623) projected
  line L547 (114.3108, -23.0623) -> (108.3108, -23.0623) projected
  line L548 (165.9108, -41.0623) -> (171.9108, -41.0623) projected
  line L549 (171.9108, -41.0623) -> (171.9108, -47.0623) projected
  line L550 (171.9108, -47.0623) -> (165.9108, -47.0623) projected
  line L551 (165.9108, -47.0623) -> (165.9108, -41.0623) projected
  line L552 (165.9108, -23.0623) -> (165.9108, -17.0623) projected
  line L553 (165.9108, -17.0623) -> (171.9108, -17.0623) projected
  line L554 (171.9108, -17.0623) -> (171.9108, -23.0623) projected
  line L555 (171.9108, -23.0623) -> (165.9108, -23.0623) projected
  line L556 (223.5108, -41.0623) -> (229.5108, -41.0623) projected
  line L557 (229.5108, -41.0623) -> (229.5108, -47.0623) projected
  line L558 (229.5108, -47.0623) -> (223.5108, -47.0623) projected
  line L559 (223.5108, -47.0623) -> (223.5108, -41.0623) projected
  line L560 (223.5108, -23.0623) -> (223.5108, -17.0623) projected
  line L561 (223.5108, -17.0623) -> (229.5108, -17.0623) projected
  line L562 (229.5108, -17.0623) -> (229.5108, -23.0623) projected
  line L563 (229.5108, -23.0623) -> (223.5108, -23.0623) projected
  line L564 (281.1108, -41.0623) -> (287.1108, -41.0623) projected
  line L565 (287.1108, -41.0623) -> (287.1108, -47.0623) projected
  line L566 (287.1108, -47.0623) -> (281.1108, -47.0623) projected
  line L567 (281.1108, -47.0623) -> (281.1108, -41.0623) projected
  line L568 (281.1108, -23.0623) -> (281.1108, -17.0623) projected
  line L569 (281.1108, -17.0623) -> (287.1108, -17.0623) projected
  line L570 (287.1108, -17.0623) -> (287.1108, -23.0623) projected
  line L571 (287.1108, -23.0623) -> (281.1108, -23.0623) projected
  point P0 (0, 0)
extrude "Extrusion1" add sketch "Sketch1" along normal mid plane 12 contours L238 L239 L240 L241 | L528 L529 L530 L531
sketch "Sketch2" plane through (-6.8892, 27.9377, 6) normal (0, -1, 0) x (1, 0, 0)
  line L0 (0, 0) -> (6, 0) projected
  line L1 (0, 0) -> (6, 0)
  line L2 (6, 0) -> (6, -6)
  line L3 (6, -6) -> (0, -6)
  line L4 (0, -6) -> (0, 0)
  point P0 (6.8892, -6)
  dimension "d2" = 6
  dimension "d3" = 6
  constraints: 8 end point, 2 parallel, 1 horizontal, 1 perpendicular
  measures "d2" distance of L2.end L3.end
  measures "d3" distance of L1.end L2.end
extrude "Extrusion2" add sketch "Sketch2" along normal up to next
sketch "Sketch4" plane through (0, 0, 6) normal (0, 0, 1) x (1, 0, 0)
  line L0 (-6.8892, 27.9377) -> (-6.8892, -17.0623) projected
  line L1 (-0.8892, 27.9377) -> (-0.8892, -17.0623) projected
  line L2 (-6.8892, -5.0623) -> (-0.8892, -5.0623)
  line L3 (-0.8892, -5.0623) -> (-0.8892, 15.9377)
  line L4 (-0.8892, 15.9377) -> (-6.8892, 15.9377)
  line L5 (-6.8892, 15.9377) -> (-6.8892, -5.0623)
  line L6 (-6.8892, -23.0623) -> (-0.8892, -23.0623) projected
  line L7 (-0.8892, 33.9377) -> (-6.8892, 33.9377) projected
  point P0 (0, 0)
  point P1 (-3.8892, -5.0623)
  dimension "d8" = 18
  dimension "d9" = 18
  constraints: 8 end point, 2 parallel, 2 point on line, 1 horizontal, 1 midpoint, 1 perpendicular
  measures "d8" distance from line of L6 point (-3.889, -5.062)
  measures "d9" distance between parallel lines of L7 L4
extrude "Extrusion3" add sketch "Sketch4" along normal blind 114
sketch "Sketch5" plane through (-6.8892, 15.9377, 6) normal (0, 1, 0) x (1, 0, 0)
  line L0 (0, 0) -> (0, -114) projected
  line L1 (6, 0) -> (6, -114) projected
  line L2 (0, -108) -> (6, -108)
  line L3 (6, -108) -> (6, -102)
  line L4 (6, -102) -> (0, -102)
  line L5 (0, -102) -> (0, -108)
  line L6 (6, -114) -> (0, -114) projected
  point P0 (6.8892, 6)
  point P1 (0, -102)
  dimension "d12" = 6
  dimension "d13" = 6
  constraints: 8 end point, 2 parallel, 2 point on line, 1 horizontal, 1 perpendicular
  measures "d12" distance between parallel lines of L6 L2
  measures "d13" distance between parallel lines of L4 L2
sketch "Sketch6" plane through (-6.8892, -5.0623, 6) normal (0, -1, 0) x (1, 0, 0)
  line L0 (6, 0) -> (6, 114) projected
  line L1 (0, 0) -> (0, 114) projected
  line L2 (6, 108) -> (0, 108)
  line L3 (0, 108) -> (0, 102)
  line L4 (0, 102) -> (6, 102)
  line L5 (6, 102) -> (6, 108)
  line L6 (0, 114) -> (6, 114) projected
  point P0 (6.8892, -6)
  point P1 (0, 108)
  dimension "d14" = 6
  dimension "d15" = 6
  constraints: 8 end point, 2 parallel, 2 point on line, 1 horizontal, 1 perpendicular
  measures "d14" distance of L3.end L2.end
  measures "d15" distance between parallel lines of L6 L2
extrude "Extrusion4" add sketch "Sketch6" along normal blind 24 contours L4 L1 L2 L0
extrude "Extrusion5" add sketch "Sketch5" along normal blind 24 contours L4 L1 L2 L0
sketch "Sketch7" plane through (-6.8892, 15.9377, 114) normal (0, 0, 1) x (1, 0, 0)
  line L0 (0, -21) -> (0, -39) projected
  line L1 (6, -39) -> (6, -21) projected
  line L2 (0, -21) -> (6, -21)
  line L3 (6, -21) -> (6, -27)
  line L4 (6, -27) -> (0, -27)
  line L5 (0, -27) -> (0, -21)
  line L6 (0, -27) -> (6, -27)
  line L7 (6, -27) -> (6, -33)
  line L8 (6, -33) -> (0, -33)
  line L9 (0, -33) -> (0, -27)
  line L10 (0, -33) -> (6, -33)
  line L11 (6, -33) -> (6, -39)
  line L12 (6, -39) -> (0, -39)
  line L13 (0, -39) -> (0, -33)
  line L14 (0, -39) -> (6, -39)
  line L15 (6, -39) -> (6, -45)
  line L16 (6, -45) -> (0, -45)
  line L17 (0, -45) -> (0, -39)
  line L18 (0, 18) -> (0, 0) projected
  line L19 (0, 0) -> (6, 0)
  line L20 (6, 0) -> (6, 6)
  line L21 (6, 6) -> (0, 6)
  line L22 (0, 6) -> (0, 0)
  line L23 (6, 12) -> (0, 12) projected
  line L24 (0, 6) -> (6, 6)
  line L25 (6, 6) -> (6, 12)
  line L26 (6, 12) -> (0, 12)
  line L27 (0, 12) -> (0, 6)
  line L28 (0, 12) -> (6, 12)
  line L29 (6, 12) -> (6, 18)
  line L30 (6, 18) -> (0, 18)
  line L31 (0, 18) -> (0, 12)
  line L32 (0, 18) -> (6, 18)
  line L33 (6, 18) -> (6, 24)
  line L34 (6, 24) -> (0, 24)
  line L35 (0, 24) -> (0, 18)
  point P0 (6.8892, -15.9377)
  point P1 (6, 6)
  point P2 (0, 6)
  dimension "d20" = 6
  dimension "d21" = 6
  dimension "d22" = 6
  dimension "d23" = 6
  dimension "d24" = 6
  dimension "d25" = 6
  dimension "d26" = 6
  dimension "d27" = 6
  dimension "d28" = 6
  dimension "d29" = 6
  dimension "d30" = 6
  dimension "d31" = 6
  dimension "d32" = 6
  dimension "d33" = 6
  dimension "d34" = 6
  constraints: 64 end point, 16 parallel, 8 horizontal, 8 perpendicular, 1 point on line
  measures "d20" distance of L2.end L3.end
  measures "d21" distance of L7.end L8.end
  measures "d22" distance of L6.end L7.end
  measures "d23" distance of L1.start L12.end
  measures "d24" distance of L10.end L1.start
  measures "d25" distance of L15.end L16.end
  measures "d26" distance of L14.end L15.end
  measures "d27" distance of L21.end L20.end
  measures "d28" distance of L20.end L19.end
  measures "d29" distance of L26.end L23.start
  measures "d30" distance of L23.start L24.end
  measures "d31" distance of L30.end L29.end
  measures "d32" distance of L29.end L28.end
  measures "d33" distance of L34.end L33.end
  measures "d34" distance of L33.end L32.end
extrude "Extrusion6" add sketch "Sketch7" along normal blind 6 contours L4 L1 L8 L0 | L12 L15 L16 L17 | L35 L34 L33 L30 | L23 L25 L21 L18
equation "\"d9\" = d8"
body "Solid1"
